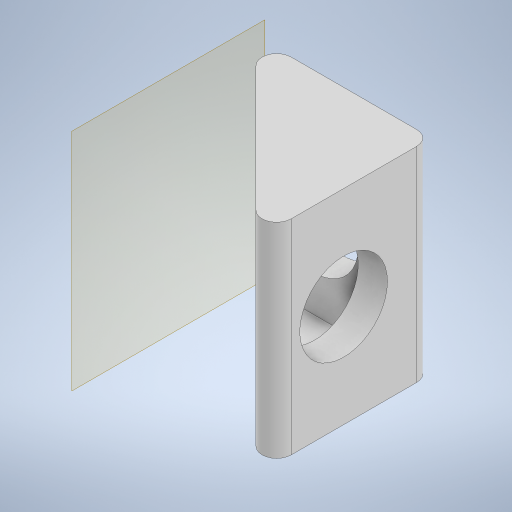
# Autodesk Inventor part: bracket
Saved by Autodesk Inventor 2023 (Build 270158000, 158)
## iProperties
Created: 2022-11-19
Part Number: bracket
Material: Generic
Document SubType Name: Modeling
Designer: samlo
Density: 1 g/cm^3
Appearance: Default
Author: samlo
Autodesk Inventor part; units mm, degrees
ref_plane "YZ Plane" through (0, 0, 0) normal (1, 0, 0) x (0, 1, 0)
ref_plane "XZ Plane" through (0, 0, 0) normal (0, 1, 0) x (-1, 0, 0)
ref_plane "XY Plane" through (0, 0, 0) normal (0, 0, 1) x (1, 0, 0)
sketch "Sketch1" plane through (0, 0, 0) normal (0, 1, 0) x (-1, 0, 0)
  line L0 (0, 0) -> (0, -6)
  line L1 (0, -6) -> (6, -6)
  line L2 (6, -6) -> (0, 0)
  dimension "d0" = 6
  dimension "d1" = 6
  constraints: 6 end point, 1 perpendicular, 1 vertical
  measures "d0" distance of L0.end L1.end
  measures "d1" distance of L0.start L0.end
extrude "Extrusion1" add sketch "Sketch1" along normal blind 7
ref_plane "Work Plane1" through (-6, 0, 0) normal (1, 0, 0) x (0, 0, -1)
fillet "Fillet1" radius 0.5 1 edges at (0, 3.5, -6)
sketch "Sketch2" plane through (-6, 0, 0) normal (1, 0, 0) x (0, 0, -1)
  line L0 (0, 0) -> (0, 7) projected
  line L1 (0, 6.25) -> (5, 6.25)
  line L2 (5, 6.25) -> (5, 0.75)
  line L3 (5, 0.75) -> (0, 0.75)
  line L4 (0, 0.75) -> (0, 6.25)
  line L5 (6, 7) -> (0, 7) projected
  point P0 (0, 0.75)
  dimension "d6" = 5.5
  dimension "d7" = 5
  dimension "d8" = 0.75
  constraints: 8 end point, 2 parallel, 1 horizontal, 1 perpendicular, 1 point on line
  measures "d6" distance of L1.end L2.end
  measures "d7" distance of L1.start L1.end
  measures "d8" distance between parallel lines of L5 L1
extrude "Extrusion2" cut sketch "Sketch2" along normal blind 5
sketch "Sketch3" plane through (-1, 0, 0) normal (-1, 0, 0) x (0, 0, 1)
  circle A0 centre (-3, 3.5) radius 1.5
  line L0 (-6, 0) -> (0, 0) projected
  dimension "d11" = 3
  dimension "d12" = 3.5
  dimension "d13" = 3
  constraints: 1 centre point
  measures "d11" diameter of A0
  measures "d12" distance from line of L0 A0.centre
  measures "d13" horizontal distance of L0.end A0.centre
extrude "Extrusion3" cut sketch "Sketch3" against normal blind 5
sketch "Sketch4" plane through (-5, 0.75, -5) normal (0, 0, 1) x (1, 0, 0)
  circle A0 centre (2, 2.75) radius 1.5
  line L0 (-1, 7.65) -> (-1, -2.15) projected
  line L1 (-1, -0.75) -> (5, -0.75) projected
  dimension "d16" = 3
  dimension "d17" = 3
  dimension "d18" = 3.5
  constraints: 1 centre point
  measures "d16" diameter of A0
  measures "d17" distance from line of L0 A0.centre
  measures "d18" distance from line of L1 A0.centre
extrude "Extrusion4" cut sketch "Sketch4" against normal blind 5
fillet "Fillet2" radius 0.5 1 edges at (-6, 3.5, -6)
fillet "Fillet3" radius 0.5 1 edges at (0, 3.5, 0)
body "Solid1"
